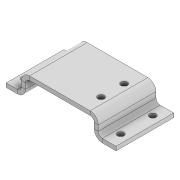
# Autodesk Inventor part: PlacaActuadorAvance
Saved by Autodesk Inventor 2021 (Build 250183000, 183)
## iProperties
Created: 2021-08-23
Part Number: PlacaActuadorAvance
Material: Generic
Document SubType Name: Sheet Metal
Designer: Santiago Suárez
Density: 1 g/cm^3
Sheet Metal Rule: Default_mm
Appearance: Default
Author: Santiago Suárez
Autodesk Inventor part; units mm, degrees
ref_plane "YZ Plane" through (0, 0, 0) normal (1, 0, 0) x (0, 1, 0)
ref_plane "XZ Plane" through (0, 0, 0) normal (0, 1, 0) x (-1, 0, 0)
ref_plane "XY Plane" through (0, 0, 0) normal (0, 0, 1) x (1, 0, 0)
sketch "Sketch1" plane through (0, 0, 0) normal (0, 1, 0) x (-1, 0, 0)
  line L0 (60, 45) -> (-60, 45)
  line L1 (-60, 45) -> (-60, -45)
  line L2 (-60, -45) -> (60, -45)
  line L3 (60, -45) -> (60, 45)
  point P0 (0, 0)
  point P1 (0, 0)
  dimension "d0" = 120
  dimension "d1" = 60
  dimension "d2" = 90
  dimension "d3" = 45
  measures "d0" distance of L0.start L0.end
  measures "d1" distance from line of L3 point (0, 0)
  measures "d2" distance of L2.end L0.start
  measures "d3" distance from line of L0 point (0, 0)
extrude "Plate1" add sketch "Sketch1" along normal blind 6.35
sketch "Sketch2" plane through (-53.65, 6.35, 45) normal (-1, 0, 0) x (0, 1, 0)
  line L0 (0, -90) -> (0, 0)
  line L1 (0, 0) -> (-34, 0)
  line L2 (-34, 0) -> (-34, -90)
  line L3 (-34, -90) -> (0, -90)
  constraints: 6 end point, 1 horizontal, 1 perpendicular, 1 vertical
edge flange "Flange1" height 34 angle 90 thickness 6.35 bend radius 6.35 thickness toward (-1, 0, 0) relief straight relief width 6.35 relief depth 3.175 edges at (-60, 6.35, 0) wall of the first edge with corners at (-53.65, 6.35, -45) (-53.65, 6.35, 45) (-53.65, -27.65, 45) (-53.65, -27.65, -45)
bend "Bend1"
corner "Corner1"
sketch "Sketch4" plane through (-53.65, -21.3, -45) normal (0, -1, 0) x (-1, 0, 0)
  line L0 (0, 90) -> (0, 0)
  line L1 (0, 0) -> (30, 0)
  line L2 (30, 0) -> (30, 90)
  line L3 (30, 90) -> (0, 90)
  constraints: 6 end point, 1 horizontal, 1 perpendicular, 1 vertical
edge flange "Flange3" height 30 angle 90 thickness 6.35 bend radius 6.35 thickness toward (0, -1, 0) relief straight relief width 6.35 relief depth 3.175 edges at (-53.65, -27.65, 0) wall of the first edge with corners at (-53.65, -21.3, 45) (-53.65, -21.3, -45) (-83.65, -21.3, -45) (-83.65, -21.3, 45)
bend "Bend3"
corner "Corner3"
sketch "Sketch5" plane through (53.65, 6.35, 45) normal (1, 0, 0) x (0, 1, 0)
  line L0 (0, -90) -> (0, 0)
  line L1 (0, 0) -> (-34, 0)
  line L2 (-34, 0) -> (-34, -90)
  line L3 (-34, -90) -> (0, -90)
  constraints: 6 end point, 1 horizontal, 1 perpendicular, 1 vertical
edge flange "Flange4" height 34 angle 90 thickness 6.35 bend radius 6.35 thickness toward (1, 0, 0) relief straight relief width 6.35 relief depth 3.175 edges at (60, 0, 0) wall of the first edge with corners at (53.65, 6.35, -45) (53.65, 6.35, 45) (53.65, -27.65, 45) (53.65, -27.65, -45)
bend "Bend4"
corner "Corner4"
sketch "Sketch6" plane through (53.65, -21.3, 45) normal (0, -1, 0) x (-1, 0, 0)
  line L0 (0, -90) -> (0, 0)
  line L1 (0, 0) -> (-34, 0)
  line L2 (-34, 0) -> (-34, -90)
  line L3 (-34, -90) -> (0, -90)
  constraints: 6 end point, 1 horizontal, 1 perpendicular, 1 vertical
edge flange "Flange5" height 34 angle 90 thickness 6.35 bend radius 6.35 thickness toward (0, -1, 0) relief straight relief width 6.35 relief depth 3.175 edges at (53.65, -27.65, 0) wall of the first edge with corners at (53.65, -21.3, -45) (53.65, -21.3, 45) (87.65, -21.3, 45) (87.65, -21.3, -45)
bend "Bend5"
corner "Corner5"
sketch "Sketch7" plane through (0, 6.35, 0) normal (0, 1, 0) x (1, 0, 0)
  line L0 (37.3, 18) -> (37.3, -18)
  line L1 (47.3, -45) -> (47.3, 45) projected
  point P0 (0, 0)
  dimension "d55" = 36
  dimension "d56" = 18
  dimension "d57" = 10
  constraints: 2 coincident, 2 end point, 1 vertical
  measures "d55" distance of L0.start L0.end
  measures "d56" vertical distance of point (0, 0) L0.start
  measures "d57" distance between parallel lines of L1 L0
hole "Hole1" at (37.3, 6.35, -18) at (37.3, 6.35, 18) direction (0, -1, 0) diameter 10 depth 6.35
sketch "Sketch8" plane through (-83.65, -21.3, 45) normal (0, 1, 0) x (1, 0, 0)
  line L0 (17.3, 0) -> (0, 0) projected
  line L1 (8.65, 0) -> (8.65, 90)
  line L2 (0, 90) -> (17.3, 90) projected
  line L3 (0, 0) -> (0, 90) projected
  line L4 (0, 20) -> (17.3, 20)
  line L5 (17.3, 0) -> (17.3, 90) projected
  line L6 (0, 70) -> (17.3, 70)
  point P0 (83.65, 45)
  point P1 (8.65, 20)
  point P2 (8.65, 70)
  dimension "d65" = 20
  dimension "d66" = 20
  constraints: 6 end point, 4 midpoint, 4 point on line, 1 horizontal, 1 perpendicular
  measures "d65" distance between parallel lines of L2 L6
  measures "d66" distance between parallel lines of L0 L4
hole "Hole2" at (-75, -21.3, 25) at (-75, -21.3, -25) direction (0, -1, 0) diameter 10 depth 6.35
mirror "Mirror1" about plane through (0, 0, 0) normal (1, 0, 0) of "Hole2"
unfold all bends "Unfold1" k factor 0.44 fixed face at (-20.6584, 6.35, -5.409)
refold all bends "Refold1"
equation "\"d56\" = 0.5 * d55"
equation "\"d63\" = Thickness"
equation "\"d72\" = Thickness"
equation "\"d4\" = Thickness"
equation "\"d5\" = BendReliefWidth"
equation "\"d6\" = BendReliefDepth"
equation "\"d7\" = MinimumRemnant"
equation "\"d8\" = TransitionRadius"
equation "\"d11\" = BendRadius"
equation "\"d12\" = CornerReliefSize"
equation "\"d13\" = GapSize"
equation "\"d14\" = JacobiRadiusSize"
equation "\"d25\" = BendReliefWidth"
equation "\"d26\" = BendReliefDepth"
equation "\"d27\" = MinimumRemnant"
equation "\"d28\" = TransitionRadius"
equation "\"d31\" = BendRadius"
equation "\"d32\" = CornerReliefSize"
equation "\"d33\" = GapSize"
equation "\"d34\" = JacobiRadiusSize"
equation "\"d35\" = BendReliefWidth"
equation "\"d36\" = BendReliefDepth"
equation "\"d37\" = MinimumRemnant"
equation "\"d38\" = TransitionRadius"
equation "\"d41\" = BendRadius"
equation "\"d42\" = CornerReliefSize"
equation "\"d43\" = GapSize"
equation "\"d44\" = JacobiRadiusSize"
equation "\"d45\" = BendReliefWidth"
equation "\"d46\" = BendReliefDepth"
equation "\"d47\" = MinimumRemnant"
equation "\"d48\" = TransitionRadius"
equation "\"d51\" = BendRadius"
equation "\"d52\" = CornerReliefSize"
equation "\"d53\" = GapSize"
equation "\"d54\" = JacobiRadiusSize"
equation "\"d1\" = 0.5 * d0"
equation "\"d3\" = 0.5 * d2"
equation "\"BendRadius\" = Thickness"
equation "\"BendReliefWidth\" = Thickness"
equation "\"BendReliefDepth\" = 0.5 * Thickness"
equation "\"CornerReliefSize\" = 4 * Thickness"
equation "\"MinimumRemnant\" = 2 * Thickness"
equation "\"TransitionRadius\" = BendRadius"
equation "\"JacobiRadiusSize\" = BendRadius"
equation "\"GapSize\" = Thickness"
equation "\"Thickness\" = 6.35"
body "Solid1"
